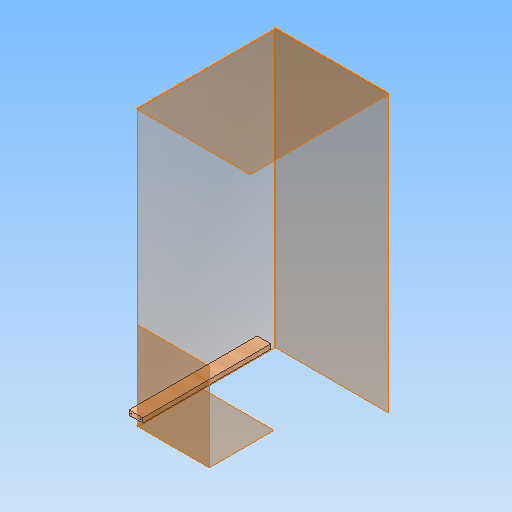
# Autodesk Inventor part: Top_Reinforcement 2
Saved by Autodesk Inventor 2018.1 (Build 221171000, 171)
## iProperties
Created: 2019-03-15
Part Number: Top_Reinforcement 2
Material: Wood (Birch)
Document SubType Name: Modeling
Designer: James
Density: 0.55 g/cm^3
Appearance: Birch - Natural Polished
Author: James
Autodesk Inventor part; units mm, degrees
ref_plane "YZ Plane" through (0, 0, 0) normal (1, 0, 0) x (0, 1, 0)
ref_plane "XZ Plane" through (0, 0, 0) normal (0, 1, 0) x (-1, 0, 0)
ref_plane "XY Plane" through (0, 0, 0) normal (0, 0, 1) x (1, 0, 0)
derived "Top_Skeleton.ipt"
ref_plane "Work Plane1" through (0, 0, 0) normal (0, 0, 1) x (1, 0, 0)
ref_plane "Work Plane2" through (0, 0, 0) normal (0, 1, 0) x (-1, 0, 0)
ref_plane "Work Plane3" through (0, 0, 0) normal (1, 0, 0) x (0, 1, 0)
ref_plane "Work Plane4" through (0, 3000, 0) normal (0, 1, 0) x (-1, 0, 0)
ref_plane "Work Plane5" through (0, 0, -1500) normal (0, 0, 1) x (1, 0, 0)
sketch "Sketch2" plane through (0, 0, 0) normal (1, 0, 0) x (0, 1, 0)
  line L0 (0, -50) -> (50, -50)
  line L1 (50, -50) -> (50, -1450)
  line L2 (50, -1450) -> (0, -1450)
  line L3 (0, -1450) -> (0, -50)
  line L4 (-10, 0) -> (60, 0) projected
  line L5 (-10, -1500) -> (60, -1500) projected
  line L6 (0, 290) -> (0, -1740) projected
  point P0 (0, 0)
  dimension "d1" = 50
  dimension "d2" = 50
  dimension "d3" = 50
  constraints: 8 end point, 2 parallel, 1 horizontal, 1 perpendicular, 1 point on line
  measures "d1" distance between parallel lines of L0 L4
  measures "d2" distance between parallel lines of L2 L5
  measures "d3" distance of L1.end L2.end
extrude "Extrusion1" add sketch "Sketch2" against normal blind 150
sketch "Sketch3" plane through (0, 0, -50) normal (0, 0, 1) x (1, 0, 0)
  line L0 (0, 50) -> (-150, 50) projected
  line L1 (0, 0) -> (-150, 0) projected
  line L2 (-150, 0) -> (-150, 50) projected
  line L3 (0, 60) -> (0, -10) projected
  point P0 (-125, 25)
  point P1 (-25, 25)
  dimension "d6" = 25
  dimension "d7" = 25
  dimension "d8" = 25
  dimension "d9" = 25
  constraints: 1 horizontal alignment
  measures "d6" distance from line of point (-125, 25) L0
  measures "d7" distance from line of L1 point (-125, 25)
  measures "d8" distance from line of L2 point (-125, 25)
  measures "d9" distance from line of L3 point (-25, 25)
hole "Hole1" at (-125, 25, -50) at (-25, 25, -50) direction (0, 0, -1) diameter 10.592 depth 35.169 tip angle 118 thread size "1/2-13 UNC" class "2B" standard "ANSI Unified Screw Threads"
ref_plane "Work Plane6" through (0, 0, -750) normal (0, 0, 1) x (1, 0, 0)
mirror "Mirror1" about plane through (0, 0, -750) normal (0, 0, 1) of "Hole1"
equation "\"d2\" = d1"
equation "\"d6\" = d7"
equation "\"d9\" = d8"
body "Solid1"
